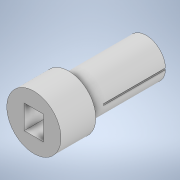
# Autodesk Inventor part: Magnethalter
Saved by Autodesk Inventor 2021 (Build 250183000, 183)
## iProperties
Created: 2024-03-24
Part Number: Magnethalter
Material: Generic
Document SubType Name: Modeling
Designer: Lukas
Density: 1 g/cm^3
Appearance: Default
Author: Lukas
Autodesk Inventor part; units mm, degrees
ref_plane "YZ Plane" through (0, 0, 0) normal (1, 0, 0) x (0, 1, 0)
ref_plane "XZ Plane" through (0, 0, 0) normal (0, 1, 0) x (-1, 0, 0)
ref_plane "XY Plane" through (0, 0, 0) normal (0, 0, 1) x (1, 0, 0)
sketch "Sketch1" plane through (0, 0, 0) normal (0, 0, 1) x (1, 0, 0)
  circle A0 centre (0, 0) radius 2.5
  dimension "d0" = 5
  constraints: 1 centre point, 1 coincident
  measures "d0" diameter of A0
extrude "Extrusion1" add sketch "Sketch1" along normal blind 10
sketch "Sketch2" plane through (0, 0, 10) normal (0, 0, 1) x (1, 0, 0)
  circle A0 centre (0, 0) radius 3.5
  dimension "d3" = 7
  constraints: 1 centre point, 1 coincident
  measures "d3" diameter of A0
extrude "Extrusion2" add sketch "Sketch2" along normal blind 4.5
sketch "Sketch3" plane through (0, 0, 14.5) normal (0, 0, 1) x (1, 0, 0)
  line L0 (-1.25, 1.55) -> (1.25, 1.55)
  line L1 (1.25, 1.55) -> (1.25, -1.55)
  line L2 (1.25, -1.55) -> (-1.25, -1.55)
  line L3 (-1.25, -1.55) -> (-1.25, 1.55)
  point P0 (0, 0)
  point P1 (-1.25, 0)
  point P2 (0, 1.55)
  dimension "d6" = 2.5
  dimension "d7" = 3.1
  constraints: 8 end point, 2 midpoint, 2 parallel, 1 horizontal, 1 horizontal alignment, 1 perpendicular, 1 vertical alignment
  measures "d6" distance of L0.start L0.end
  measures "d7" distance of L0.end L1.end
extrude "Extrusion3" cut sketch "Sketch3" against normal blind 4
sketch "Sketch4" plane through (0, 0, 0) normal (0, 0, -1) x (-1, 0, 0)
  circle A0 centre (0, 0) radius 0.5
  line L0 (2.5, -0.1) -> (-2.5, -0.1)
  line L1 (-2.5, -0.1) -> (-2.5, 0.1)
  line L2 (-2.5, 0.1) -> (2.5, 0.1)
  line L3 (2.5, 0.1) -> (2.5, -0.1)
  point P0 (0, -0.1)
  point P1 (2.5, 0)
  point P2 (-0.4899, 0.1)
  point P3 (-0.4899, -0.1)
  point P4 (0.4899, -0.1)
  point P5 (0.4899, 0.1)
  dimension "d10" = 1
  dimension "d11" = 5
  dimension "d12" = 0.2
  constraints: 8 end point, 2 midpoint, 2 parallel, 1 centre point, 1 coincident, 1 horizontal, 1 horizontal alignment, 1 perpendicular, 1 vertical alignment
  measures "d10" diameter of A0
  measures "d11" distance of L0.start L0.end
  measures "d12" distance of L2.end L0.start
extrude "Extrusion4" cut sketch "Sketch4" against normal blind 8
body "Solid1"
